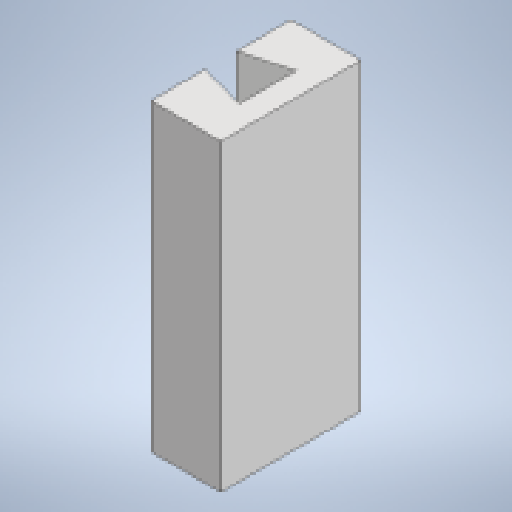
# Autodesk Inventor part: Laser_Base
Saved by Autodesk Inventor 2023 (Build 270158000, 158)
## iProperties
Created: 2024-01-06
Part Number: Laser_Base
Material: Generic
Document SubType Name: Modeling
Designer: a laptop
Density: 1 g/cm^3
Appearance: Default
Author: a laptop
Autodesk Inventor part; units mm, degrees
ref_plane "YZ Plane" through (0, 0, 0) normal (1, 0, 0) x (0, 1, 0)
ref_plane "XZ Plane" through (0, 0, 0) normal (0, 1, 0) x (-1, 0, 0)
ref_plane "XY Plane" through (0, 0, 0) normal (0, 0, 1) x (1, 0, 0)
sketch "Sketch1" plane through (0, 0, 0) normal (0, 1, 0) x (-1, 0, 0)
  line L0 (0, 0) -> (15, 0)
  line L1 (15, 0) -> (15, -11.5795)
  line L2 (15, -11.5795) -> (5, -8.9)
  line L3 (5, -8.9) -> (5, -21.1)
  line L4 (5, -21.1) -> (15, -18.4205)
  line L5 (15, -18.4205) -> (15, -30)
  line L6 (15, -30) -> (0, -30)
  line L7 (0, -30) -> (0, 0)
  point P0 (5, -15)
  dimension "d0" = 12.2
  dimension "d1" = 30
  dimension "d2" = 15
  dimension "d3" = 10
  dimension "d4" = 30
  constraints: 16 end point, 3 equal length, 2 parallel, 2 perpendicular, 1 collinear, 1 horizontal, 1 midpoint
  measures "d0" distance of L2.end L3.end
  measures "d1" distance of L6.end L0.start
  measures "d2" distance of L5.end L6.end
  measures "d3" distance from line of L5 point (5, -15)
  measures "d4" angle of L4 L2
extrude "Extrusion1" add sketch "Sketch1" along normal blind 60
sketch "Sketch2" plane through (0, 0, 0) normal (0, -1, 0) x (1, 0, 0)
  line L0 (0, -30) -> (-15, -30) projected
  line L1 (0, 0) -> (0, -30) projected
  line L2 (-15, 0) -> (0, 0) projected
  line L3 (-15, -11.5795) -> (-15, 0) projected
  line L4 (-5, -8.9) -> (-15, -11.5795) projected
  line L5 (-5, -21.1) -> (-5, -8.9) projected
  line L6 (-15, -18.4205) -> (-5, -21.1) projected
  line L7 (-15, -30) -> (-15, -18.4205) projected
  line L8 (-15, -18.4205) -> (-15, -11.5795)
  circle A0 centre (-10, -15) radius 3
  point P0 (-15, -15)
  point P1 (-10, -19.7603)
  dimension "d9" = 6
  constraints: 2 end point, 2 midpoint, 1 centre point, 1 horizontal alignment, 1 vertical alignment
  measures "d9" diameter of A0
extrude "Extrusion2" add sketch "Sketch2" along normal blind 5
body "Solid1"
